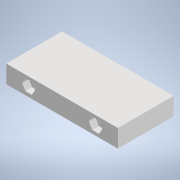
# Autodesk Inventor part: 14_base_avanti
Saved by Autodesk Inventor 2020 (Build 240168000, 168)
## iProperties
Created: 2019-10-17
Part Number: 14_base_avanti
Material: Generico
Document SubType Name: Modeling
Designer: socci
Density: 1 g/cm^3
Appearance: Default
Author: socci
Autodesk Inventor part; units mm, degrees
ref_plane "YZ Plane" through (0, 0, 0) normal (1, 0, 0) x (0, 1, 0)
ref_plane "XZ Plane" through (0, 0, 0) normal (0, 1, 0) x (-1, 0, 0)
ref_plane "XY Plane" through (0, 0, 0) normal (0, 0, 1) x (1, 0, 0)
sketch "Schizzo1" plane through (0, 0, 0) normal (0, 1, 0) x (-1, 0, 0)
  line L0 (50, -25) -> (-50, -25)
  line L1 (-50, -25) -> (-50, 25)
  line L2 (-50, 25) -> (50, 25)
  line L3 (50, 25) -> (50, -25)
  line L4 (50, -25) -> (-50, 25) construction
  line L5 (-50, -25) -> (50, 25) construction
  point P0 (0, 0)
  point P1 (0, 0)
  point P2 (0, 0)
  dimension "d0" = 50
  dimension "d9" = 100
  constraints: 12 end point, 3 midpoint, 2 parallel, 1 coincident, 1 horizontal, 1 perpendicular
  measures "d0" distance of L0.end L1.end
  measures "d9" distance of L1.end L2.end
extrude "Estrusione1" add sketch "Schizzo1" along normal blind 16
sketch "Schizzo2" plane through (0, 0, 0) normal (0, -1, 0) x (1, 0, 0)
  circle A0 centre (0, -25) radius 9.5
  line L0 (50, -25) -> (-50, -25) projected
  point P0 (0, 0)
  dimension "d3" = 19
  constraints: 1 centre point, 1 coincident, 1 midpoint
  measures "d3" diameter of A0
extrude "Estrusione2" cut sketch "Schizzo2" against normal blind 4
sketch "Schizzo3" plane through (0, 4, 0) normal (0, -1, 0) x (1, 0, 0)
  circle A0 centre (0, -25) radius 6
  line L0 (9.5, -25) -> (-9.5, -25) projected
  point P0 (0, 0)
  dimension "d6" = 12
  constraints: 1 centre point, 1 coincident, 1 midpoint
  measures "d6" diameter of A0
extrude "Estrusione3" cut sketch "Schizzo3" against normal blind 10
sketch "Schizzo4" plane through (-50, 0, 25) normal (0, 0, 1) x (1, 0, 0)
  line L0 (50, 0) -> (50, 8)
  line L1 (50, 0) -> (58, 0) construction
  line L2 (50, 8) -> (20, 8)
  line L3 (50, 8) -> (80, 8)
  line L4 (50, 8) -> (80, 8) construction
  dimension "d10" = 8
  dimension "d11" = 90
  dimension "d12" = 30
  dimension "d13" = 90
  dimension "d14" = 30
  dimension "d15" = 0
  constraints: 10 end point, 3 horizontal, 2 equal length, 1 perpendicular, 1 vertical
  measures "d10" distance of L0.start L0.end
  measures "d11" angle of L1 L0
  measures "d12" distance of L0.end L2.end
  measures "d13" angle of L2 L0
  measures "d14" distance of L0.end L3.end
  measures "d15" distance between parallel lines of L3 L4
hole "Foro1" at (30, 8, 25) at (-30, 8, 25) direction (0, 0, -1) diameter 6.6 end through all clearance for "Bullone a testa esagonale" size "M6" standard "ANSI - Profilo M Metrico"
sketch "Schizzo5" plane through (-50, 0, 25) normal (0, 0, 1) x (1, 0, 0)
  circle A0 centre (80, 8) radius 3.3 projected
  circle A1 centre (80, 8) radius 5
  circle A2 centre (20, 8.2293) radius 5
  line L0 (17.1132, 3.2293) -> (14.2265, 8.2293)
  line L1 (14.2265, 8.2293) -> (17.1132, 13.2293)
  line L2 (17.1132, 13.2293) -> (22.8868, 13.2293)
  line L3 (22.8868, 13.2293) -> (25.7735, 8.2293)
  line L4 (25.7735, 8.2293) -> (22.8868, 3.2293)
  line L5 (22.8868, 3.2293) -> (17.1132, 3.2293)
  line L6 (76.9809, 3) -> (73.9618, 8.2293)
  line L7 (73.9618, 8.2293) -> (76.9809, 13.4586)
  line L8 (76.9809, 13.4586) -> (83.0191, 13.4586)
  line L9 (83.0191, 13.4586) -> (86.0382, 8.2293)
  line L10 (86.0382, 8.2293) -> (83.0191, 3)
  line L11 (83.0191, 3) -> (76.9809, 3)
  point P0 (50, 0)
  point P1 (20, 3.2293)
  point P2 (80, 8.2293)
  point P3 (80, 3)
  dimension "d24" = 10
  dimension "d25" = 10
  constraints: 24 end point, 2 coincident, 2 midpoint, 2 vertical alignment, 30 other
extrude "Estrusione4" cut sketch "Schizzo5" against normal blind 6 contours A0 | A1 | L11 L6 L7 L8 L9 L10 | A2 | A2 L3 L4 | A2 L2 L3 | L4 L5 A2 | A2 L1 L2 | L5 L0 A2 | A2 L0 L1
